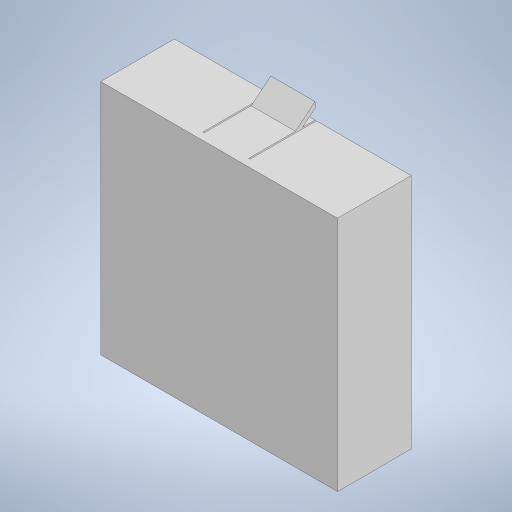
# Autodesk Inventor part: Part_6_lid
Saved by Autodesk Inventor 2023 (Build 270158000, 158)
## iProperties
Created: 2023-10-25
Part Number: Part_6_lid
Material: Generic
Document SubType Name: Modeling
Designer: zskus
Density: 1 g/cm^3
Appearance: Default
Author: zskus
Autodesk Inventor part; units mm, degrees
ref_plane "YZ Plane" through (0, 0, 0) normal (1, 0, 0) x (0, 1, 0)
ref_plane "XZ Plane" through (0, 0, 0) normal (0, 1, 0) x (-1, 0, 0)
sketch "Sketch1" plane through (0, 0, 0) normal (0, 0, 1) x (1, 0, 0)
  line L0 (-38.227, 38.227) -> (38.227, 38.227)
  line L1 (38.227, 38.227) -> (38.227, -38.227)
  line L2 (38.227, -38.227) -> (-38.227, -38.227)
  line L3 (-38.227, -38.227) -> (-38.227, 38.227)
  point P0 (0, 0)
  dimension "d0" = 76.454
  dimension "d1" = 76.454
  dimension "d2" = 38.227
  dimension "d3" = 38.227
  constraints: 8 end point, 2 parallel, 1 horizontal, 1 perpendicular
  measures "d0" distance of L0.end L1.end
  measures "d1" distance of L0.start L0.end
  measures "d2" distance from line of point (0, 0) L1
  measures "d3" distance from line of L0 point (0, 0)
extrude "Extrusion1" add sketch "Sketch1" along normal blind 2.54
sketch "Sketch2" plane through (0, 0, 2.54) normal (0, 0, 1) x (1, 0, 0)
  line L0 (-38.227, -38.227) -> (38.227, -38.227) projected
  line L1 (38.227, -38.227) -> (38.227, 38.227) projected
  line L2 (38.227, 38.227) -> (-38.227, 38.227) projected
  line L3 (-38.227, 38.227) -> (-38.227, -38.227) projected
  line L4 (-40.767, 40.767) -> (40.767, 40.767)
  line L5 (40.767, 40.767) -> (40.767, -40.767)
  line L6 (40.767, -40.767) -> (-40.767, -40.767)
  line L7 (-40.767, -40.767) -> (-40.767, 40.767)
  point P0 (0, 0)
  dimension "d6" = 2.54
  constraints: 8 end point, 3 other
  measures "d6" distance between parallel lines of L2 L4
extrude "Extrusion2" add sketch "Sketch2" against normal blind 25.4
sketch "Sketch3" plane through (-40.767, 40.767, 2.54) normal (0, 1, 0) x (1, 0, 0)
  line L0 (81.534, 0) -> (0, 0) projected
  line L1 (81.534, 0) -> (81.534, 25.4) projected
  line L2 (0, 25.4) -> (81.534, 25.4) projected
  line L3 (0, 0) -> (0, 25.4) projected
  line L4 (78.994, 2.54) -> (2.54, 2.54) projected
  line L5 (2.54, 2.54) -> (2.54, 25.4) projected
  line L6 (78.994, 2.54) -> (78.994, 25.4) projected
  line L7 (33.147, 2.54) -> (32.639, 2.54)
  line L8 (32.639, 2.54) -> (32.639, 25.4)
  line L9 (32.639, 25.4) -> (33.147, 25.4)
  line L10 (33.147, 25.4) -> (33.147, 2.54)
  line L11 (78.994, 25.4) -> (2.54, 25.4) projected
  line L12 (48.387, 2.54) -> (48.895, 2.54)
  line L13 (48.895, 2.54) -> (48.895, 25.4)
  line L14 (48.895, 25.4) -> (48.387, 25.4)
  line L15 (48.387, 25.4) -> (48.387, 2.54)
  point P0 (40.767, 2.54)
  point P1 (40.767, 2.54)
  dimension "d9" = 15.24
  dimension "d10" = 7.62
  dimension "d11" = 0.508
  dimension "d12" = 0.508
  constraints: 16 end point, 4 parallel, 4 point on line, 2 horizontal, 2 perpendicular, 1 midpoint
  measures "d9" distance between parallel lines of L15 L10
  measures "d10" distance from line of point (40.767, 2.54) L15
  measures "d11" distance between parallel lines of L15 L13
  measures "d12" distance between parallel lines of L10 L8
extrude "Extrusion3" cut sketch "Sketch3" against normal blind 25.4 contours L13 L4 L15 L2 | L2 L10 L4 L8
ref_plane "Work Plane1" through (5.08, 40.767, 0) normal (1, 0, 0) x (0, 0, -1)
sketch "Sketch6" plane through (5.08, 40.767, 0) normal (1, 0, 0) x (0, 0, -1)
  line L0 (0, -2.54) -> (22.86, -2.54) projected
  line L1 (0, 0) -> (0, -2.54) projected
  line L2 (22.86, 0) -> (0, 0) projected
  line L3 (22.86, -2.54) -> (22.86, 0) projected
  line L4 (-2.54, 0) -> (-2.54, -81.534) projected
  line L5 (-2.54, 0) -> (22.86, 0) projected
  line L6 (22.86, -81.534) -> (22.86, 0) projected
  line L7 (-2.54, -81.534) -> (22.86, -81.534) projected
  line L8 (0, -2.54) -> (0, -78.994) projected
  line L9 (0, -78.994) -> (22.86, -78.994) projected
  line L10 (22.86, -2.54) -> (22.86, -78.994) projected
  line L11 (0, -2.54) -> (22.86, -2.54) projected
  line L12 (3.2004, -2.54) -> (3.2004, -3.81)
  line L13 (3.2004, -3.81) -> (6.35, -2.54)
  point P0 (0, -40.767)
  point P1 (6.35, -2.54)
  point P2 (3.2004, -2.54)
  dimension "d20" = 3.2004
  dimension "d21" = 3.1496
  dimension "d22" = 1.27
  constraints: 4 end point, 2 point on line, 1 vertical
  measures "d20" distance between parallel lines of L8 L12
  measures "d21" distance from line of L12 L13.end
  measures "d22" distance of L12.start L12.end
extrude "Extrusion4" add sketch "Sketch6" against normal blind 10.16 contours L0 L13 L12
sketch "Sketch7" plane through (7.62, 40.767, 0) normal (1, 0, 0) x (0, 0, -1)
  line L0 (0, -2.54) -> (22.86, -2.54) projected
  line L1 (0, 0) -> (0, -2.54) projected
  line L2 (22.86, 0) -> (0, 0) projected
  line L3 (22.86, -2.54) -> (22.86, 0) projected
  line L4 (22.86, 5.5075) -> (16.1237, 0)
  line L5 (-2.54, 0) -> (22.86, 0) projected
  line L6 (18.6021, 0) -> (22.86, 3.4812)
  line L7 (22.86, 3.4812) -> (22.86, 5.5075)
  point P0 (0, -40.767)
  constraints: 6 end point, 2 point on line, 1 parallel, 1 perpendicular
extrude "Extrusion5" add sketch "Sketch7" against normal blind 15.24 contours L4 L7 L6 L2
equation "\"d2\" = 0.5 * d1"
equation "\"d3\" = 0.5 * d0"
equation "\"d10\" = 0.5 * d9"
equation "\"d12\" = d11"
body "Solid1"
